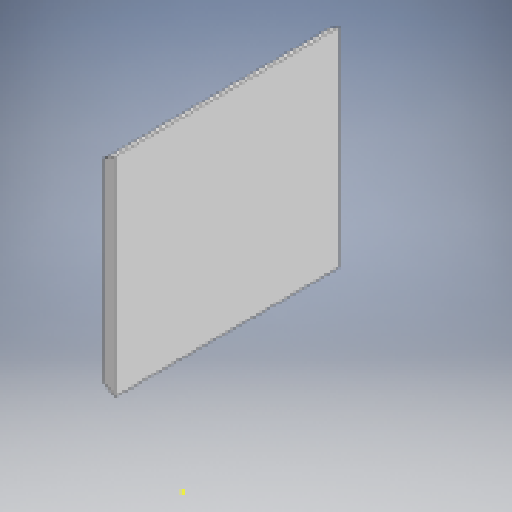
# Autodesk Inventor part: door
Saved by Autodesk Inventor 2025.2 (Build 292293000, 293)
## iProperties
Created: 2025-02-23
Part Number: door
Material: Generic
Document SubType Name: Modeling
Designer: Alex
Density: 1 g/cm^3
Appearance: Default
Author: Alex
Autodesk Inventor part; units mm, degrees
ref_plane "YZ Plane" through (0, 0, 0) normal (1, 0, 0) x (0, 1, 0)
ref_plane "XZ Plane" through (0, 0, 0) normal (0, 1, 0) x (-1, 0, 0)
ref_plane "XY Plane" through (0, 0, 0) normal (0, 0, 1) x (1, 0, 0)
sketch "Sketch1" plane through (0, 0, 0) normal (0, 0, 1) x (1, 0, 0)
  line L0 (-45, 93) -> (-45, 89.5) construction
  line L1 (-45, 89.5) -> (50, 89.5) construction
  line L2 (50, 89.5) -> (50, 96.5) construction
  line L3 (50, 96.5) -> (-50, 96.5) construction
  line L4 (-50, 96.5) -> (-50, 89.5) construction
  line L5 (-50, 89.5) -> (-45, 93) construction
  line L6 (-45, 3.5) -> (-45, 0) construction
  line L7 (-45, 0) -> (-50, 3.5) construction
  line L8 (-50, 3.5) -> (-50, -3.5) construction
  line L9 (-50, -3.5) -> (50, -3.5) construction
  line L10 (50, -3.5) -> (50, 3.5) construction
  line L11 (50, 3.5) -> (-45, 3.5) construction
  line L12 (-49.9, 89.4479) -> (-45.1, 92.8079)
  line L13 (-45.1, 92.8079) -> (-45.1, 0.1921)
  line L14 (-45.1, 0.1921) -> (-49.9, 3.5521)
  line L15 (-49.9, 3.5521) -> (-49.9, 89.4479)
  point P0 (0, 0)
  dimension "d0" = 0.1
  dimension "d1" = 0.1
  dimension "d2" = 0.1
  dimension "d3" = 0.1
  constraints: 8 end point, 1 equal length, 1 parallel
  measures "d0" distance between parallel lines of L5 L12
  measures "d1" distance between parallel lines of L0 L13
  measures "d2" distance between parallel lines of L4 L15
  measures "d3" distance between parallel lines of L7 L14
extrude "Extrusion1" add sketch "Sketch1" against normal blind 100
sketch "Sketch2" plane through (-49.9, 3.5521, -100) normal (-0.5734623, -0.8192319, 0) x (0.8192319, -0.5734623, 0)
  circle A0 centre (2.9996, 10) radius 1.3149 construction
  circle A1 centre (2.9996, 10) radius 1.125
  point P0 (42.9166, 100)
  dimension "d6" = 2.25
  constraints: 1 centre point, 1 coincident
  measures "d6" diameter of A1
extrude "Extrusion2" add sketch "Sketch2" along normal blind 0.7
fillet "Fillet1" radius 1 1 edges at (-48.7657, 1.9036, -90)
sketch "Sketch3" plane through (0, 0, -100) normal (0, 0, -1) x (-1, 0, 0)
  line L0 (50, 89.5) -> (45, 93) projected
  line L1 (45.1, 0.1921) -> (49.9, 3.5521) projected
  line L2 (49.9, 3.5521) -> (49.9, 89.4479) projected
  line L3 (49.9, 89.4479) -> (45.1, 92.8079) projected
  line L4 (45.1, 92.8079) -> (45.1, 0.1921) projected
  point P0 (0, 0)
extrude "Extrusion3" cut sketch "Sketch3" against normal blind 0.15
fillet "Fillet2" radius 1 1 edges at (-48.3643, 2.4771, -90)
body "Solid1"
